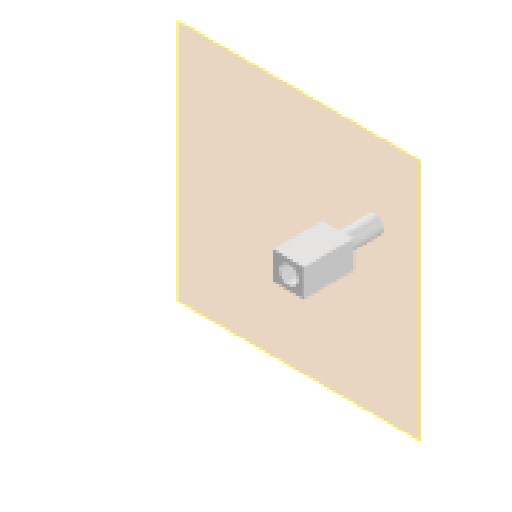
# Autodesk Inventor part: Гайка
Saved by Autodesk Inventor 2026 (Build 300175000, 175)
## iProperties
Created: 2026-04-20
Part Number: Гайка
Material: Типовые
Document SubType Name: Modeling
Designer: Artem Sannikov
Density: 1 g/cm^3
Appearance: По умолчанию
Author: Artem Sannikov
Autodesk Inventor part; units mm, degrees
ref_plane "YZ Plane" through (0, 0, 0) normal (1, 0, 0) x (0, 1, 0)
ref_plane "XZ Plane" through (0, 0, 0) normal (0, 1, 0) x (-1, 0, 0)
ref_plane "XY Plane" through (0, 0, 0) normal (0, 0, 1) x (1, 0, 0)
sketch "Эскиз1" plane through (0, 0, 0) normal (0, 0, 1) x (1, 0, 0)
  circle A0 centre (60.6218, 35) radius 7.5 projected
  circle A1 centre (60.6218, 35) radius 7
  point P0 (0, 0)
  dimension "d0" = 14
  constraints: 1 centre point, 1 coincident
  measures "d0" diameter of A1
extrude "Выдавливание1" add sketch "Эскиз1" along normal blind 29.5 contours A1
sketch "Эскиз2" plane through (60.6218, 35, 29.5) normal (0, 0, 1) x (1, 0, 0)
  line L0 (12.5, 11.1132) -> (-12.5, 11.1132)
  line L1 (-12.5, 11.1132) -> (-12.5, -11.1132)
  line L2 (-12.5, -11.1132) -> (12.5, -11.1132)
  line L3 (12.5, -11.1132) -> (12.5, 11.1132)
  line L4 (12.5, 11.1132) -> (-12.5, -11.1132) construction
  line L5 (-12.5, 11.1132) -> (12.5, -11.1132) construction
  point P0 (-60.6218, -35)
  point P1 (0, 0)
  dimension "d3" = 25
  constraints: 12 end point, 2 midpoint, 2 parallel, 1 horizontal, 1 perpendicular
  measures "d3" distance of L2.end L1.end
extrude "Выдавливание2" add sketch "Эскиз2" along normal blind 40
sketch "Эскиз3" plane through (60.6218, 35, 69.5) normal (0, 0, 1) x (1, 0, 0)
  circle A0 centre (0, 0) radius 7.5
  point P0 (-60.6218, -35)
  dimension "d6" = 15
  constraints: 1 centre point
  measures "d6" diameter of A0
extrude "Выдавливание3" cut sketch "Эскиз3" against normal blind 34.25
